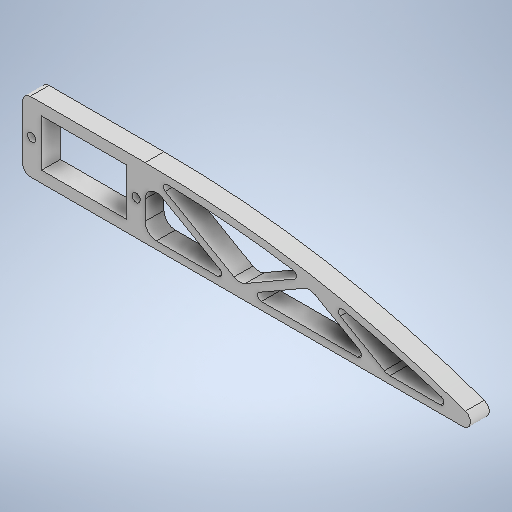
# Autodesk Inventor part: foot_v0.1
Saved by Autodesk Inventor 2025 (Build 290162000, 162)
## iProperties
Created: 2024-06-04
Part Number: foot_v0.1
Material: Generic
Document SubType Name: Modeling
Designer: sgols
Density: 1 g/cm^3
Appearance: Default
Mass: 3.42087 g
Surface Area: 39.1081 cm^2
Volume: 3.42087 cm^3
Author: sgols
Autodesk Inventor part; units mm, degrees
ref_plane "YZ Plane" through (0, 0, 0) normal (1, 0, 0) x (0, 1, 0)
ref_plane "XZ Plane" through (0, 0, 0) normal (0, 1, 0) x (-1, 0, 0)
ref_plane "XY Plane" through (0, 0, 0) normal (0, 0, 1) x (1, 0, 0)
sketch "Sketch1" plane through (0, 0, 0) normal (0, 0, 1) x (1, 0, 0)
  line L0 (0, 0) -> (32.5, 0)
  line L1 (32.5, 0) -> (32.5, 18.5)
  line L2 (32.5, 18.5) -> (0, 18.5)
  line L3 (0, 18.5) -> (0, 0)
  line L4 (5, 3) -> (27.5, 3)
  line L5 (27.5, 3) -> (27.5, 15.5)
  line L6 (27.5, 15.5) -> (5, 15.5)
  line L7 (5, 15.5) -> (5, 3)
  line L8 (27.5, 9.25) -> (32.5, 9.25) construction
  line L9 (5, 9.25) -> (0, 9.25) construction
  line L10 (16.25, 18.5) -> (16.25, 15.5) construction
  line L11 (16.25, 3) -> (16.25, 0) construction
  circle A0 centre (2.35, 9.25) radius 1.1
  circle A1 centre (30.15, 9.25) radius 1.1
  line L12 (32.5, 0) -> (120, 0)
  line L13 (120, 0) -> (120, 3)
  arc A2 (120, 3) -> (32.5, 18.5) centre (32.5, -236.2258) ccw
  arc A3 (116.873, 2) -> (32.5, 16.5) centre (32.5, -236.2258) ccw
  line L14 (116.873, 2) -> (32.5, 2)
  line L15 (32.5, 16.5) -> (57.6147, 2)
  line L16 (57.6147, 2) -> (76.1508, 12.7018)
  line L17 (76.1508, 12.7018) -> (94.6868, 2)
  line L18 (94.6868, 2) -> (102.617, 6.5785) construction
  line L19 (102.617, 6.5785) -> (94.6868, 2) construction
  line L20 (94.6868, 2) -> (94.1868, 2.866) construction
  line L21 (94.1868, 2.866) -> (102.117, 7.4445) construction
  line L22 (102.117, 7.4445) -> (102.617, 6.5785) construction
  line L23 (94.6868, 2) -> (76.1508, 12.7018)
  line L24 (76.1508, 12.7018) -> (76.6508, 13.5678)
  line L25 (76.6508, 13.5678) -> (96.6868, 2)
  line L26 (76.1508, 12.7018) -> (57.6147, 2)
  line L27 (57.6147, 2) -> (57.1147, 2.866)
  line L28 (57.1147, 2.866) -> (75.6508, 13.5678)
  line L29 (75.6508, 13.5678) -> (76.1508, 12.7018)
  line L30 (57.6147, 2) -> (32.5, 16.5)
  line L31 (32.5, 16.5) -> (33, 17.366)
  line L32 (33, 17.366) -> (58.1147, 2.866)
  line L33 (58.1147, 2.866) -> (57.6147, 2)
  line L34 (94.6868, 2) -> (95.1868, 1.134) construction
  line L35 (95.1868, 1.134) -> (103.117, 5.7125) construction
  line L36 (103.117, 5.7125) -> (103.9456, 6.1909) construction
  line L37 (76.1508, 12.7018) -> (75.6508, 11.8358)
  line L38 (75.6508, 11.8358) -> (92.6868, 2)
  line L39 (92.6868, 2) -> (94.6868, 2)
  line L40 (57.6147, 2) -> (58.1147, 1.134)
  line L41 (58.1147, 1.134) -> (76.6508, 11.8358)
  line L42 (76.6508, 11.8358) -> (76.1508, 12.7018)
  line L43 (32.5, 16.5) -> (32, 15.634)
  line L44 (32, 15.634) -> (57.1147, 1.134)
  line L45 (57.1147, 1.134) -> (57.6147, 2)
  line L46 (103.9456, 6.1909) -> (102.617, 6.5785)
  point P0 (32.5, 16.5)
  point P1 (101.2792, 6.9608)
  point P2 (94.6868, 3.1547)
  point P3 (79.0671, 12.1727)
  point P4 (74.6102, 12.967)
  point P5 (57.6147, 3.1547)
  point P6 (34.5139, 16.492)
  point P7 (32.5, 15.3453)
  point P8 (55.6147, 2)
  point P9 (59.6147, 2)
  point P10 (76.1508, 11.5471)
  point P11 (92.6868, 2)
  point P12 (96.6868, 2)
  dimension "d8" = 5
  dimension "d10" = 3
  dimension "d11" = 22.5
  dimension "d13" = 12.5
  dimension "d14" = 2.65
  dimension "d16" = 2.2
  dimension "d17" = 120
  dimension "d18" = 3
  dimension "d23" = 2
  dimension "d73" = 30
  dimension "d74" = 30
  dimension "d75" = 30
  dimension "d76" = 30
  dimension "d77" = 1
  constraints: 94 end point, 12 parallel, 8 midpoint, 8 point on line, 8 symmetric about line, 7 perpendicular, 7 point on circle, 4 centre point, 4 equal length, 3 collinear, 3 horizontal, 1 tangent, 1 vertical, 2 other
  measures "d8" distance of L8.start L8.end
  measures "d10" distance of L11.start L11.end
  measures "d11" distance between parallel lines of L5 L7
  measures "d13" distance of L4.end L5.end
  measures "d14" distance of A0.centre L9.start
  measures "d16" diameter of A0
  measures "d17" distance of L12.end L0.start
  measures "d18" distance of L12.end L13.end
  measures "d23" radial gap between concentric circles of A2 A3
  measures "d73" angle of L14 L15
  measures "d74" angle of L14 L16
  measures "d75" angle of L14 L17
  measures "d76" angle of L14 L18
  measures "d77" distance of L16.end L24.end
extrude "Extrusion1" add sketch "Sketch1" along normal mid plane 5 contours L3 L2 L1 L43 L44 L0 | L1 L14 L44 L45 L40 L41 A3 L25 L24 L29 L28 L32 L31 A2 L13 L12 | L44 L43 L1 | L1 L15 L14 L44 | L14 L45 L44 | L31 L32 A3 | A3 L32 L28 L27 L15 | L16 L37 L38 L41 L14 | L33 L32 L28 A3 L16 | L27 L28 L32 L33 | L14 L41 L40 | L24 L25 A3 | A3 L25 L14 L17 | A3 L28 L29 | L42 L41 L38 L37 | L17 L14 L38 L41 L42
fillet "Fillet3" radius 2 4 edges at (0, 18.5, 0) (0, 0, 0) (120, 0, 0) (120, 3, 0)
fillet "Fillet5" radius 3 5 edges at (76.1508, 11.5471, 0) (32.5, 15.3453, 0) (57.6147, 3.1547, 0) (96.6868, 2, 0) (32.5, 2, 0)
fillet "Fillet5" radius 1 7 edges at (116.873, 2, 0) (92.6868, 2, 0) (79.0671, 12.1727, 0) (34.5139, 16.492, 0) (74.6102, 12.967, 0) (59.6147, 2, 0) (55.6147, 2, 0)
body "Solid1"
